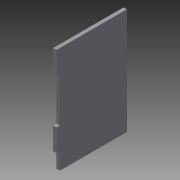
# Autodesk Inventor part: Motor support
Saved by Autodesk Inventor 2015 (Build 190159000, 159)
## iProperties
Created: 2014-11-11
Part Number: Motor support
Material: Generic
Document SubType Name: Modeling
Designer: karl
Density: 1 g/cm^3
Appearance: Default
Author: karl
Autodesk Inventor part; units mm, degrees
ref_plane "YZ Plane" through (0, 0, 0) normal (1, 0, 0) x (0, 1, 0)
ref_plane "XZ Plane" through (0, 0, 0) normal (0, 1, 0) x (-1, 0, 0)
ref_plane "XY Plane" through (0, 0, 0) normal (0, 0, 1) x (1, 0, 0)
sketch "Sketch1" plane through (0, 0, 0) normal (1, 0, 0) x (0, 1, 0)
  line L0 (-35, -47.5) -> (35, -47.5)
  line L1 (35, -47.5) -> (35, 47.5)
  line L2 (35, 47.5) -> (-35, 47.5)
  line L3 (-35, 47.5) -> (-35, -47.5)
  line L4 (-35, -47.5) -> (35, 47.5) construction
  line L5 (35, -47.5) -> (-35, 47.5) construction
  point P0 (0, 0)
  dimension "d0" = 70
  dimension "d1" = 95
  constraints: 12 end point, 2 midpoint, 2 parallel, 1 horizontal, 1 perpendicular
  measures "d0" distance of L2.end L1.end
  measures "d1" distance of L1.end L0.end
extrude "Extrusion1" add sketch "Sketch1" along normal blind 3
sketch "Sketch2" plane through (3, 0, 0) normal (1, 0, 0) x (0, 0, -1)
  line L0 (-47.5, -35) -> (47.5, -35) projected
  line L1 (32.5, -35) -> (12.5, -35)
  line L2 (12.5, -35) -> (12.5, -38)
  line L3 (12.5, -38) -> (32.5, -38)
  line L4 (32.5, -38) -> (32.5, -35)
  line L5 (-27.5, -35) -> (-47.5, -35)
  line L6 (-47.5, -35) -> (-47.5, -38)
  line L7 (-47.5, -38) -> (-27.5, -38)
  line L8 (-27.5, -38) -> (-27.5, -35)
  line L9 (47.5, -35) -> (47.5, 35) projected
  point P0 (0, 0)
  dimension "d4" = 20
  dimension "d5" = 3
  dimension "d6" = 20
  dimension "d7" = 3
  dimension "d8" = 40
  dimension "d9" = 15
  constraints: 16 end point, 4 parallel, 2 horizontal, 2 perpendicular, 2 point on line
  measures "d4" distance of L3.end L2.end
  measures "d5" distance of L2.end L1.end
  measures "d6" distance of L7.end L6.end
  measures "d7" distance of L6.end L5.end
  measures "d8" distance between parallel lines of L2 L8
  measures "d9" distance between parallel lines of L9 L4
extrude "Extrusion2" add sketch "Sketch2" against normal blind 3
sketch "Sketch3" plane through (3, 0, 0) normal (1, 0, 0) x (0, 0, -1)
  line L0 (47.5, -35) -> (47.5, 35) projected
  line L1 (47.5, 25) -> (50.5, 25)
  line L2 (50.5, 25) -> (50.5, 5)
  line L3 (50.5, 5) -> (47.5, 5)
  line L4 (47.5, 5) -> (47.5, 25)
  line L5 (47.5, 35) -> (-47.5, 35) projected
  line L6 (47.5, -15) -> (50.5, -15)
  line L7 (50.5, -15) -> (50.5, -25)
  line L8 (50.5, -25) -> (47.5, -25)
  line L9 (47.5, -25) -> (47.5, -15)
  line L10 (32.5, -35) -> (47.5, -35) projected
  point P0 (0, 0)
  dimension "d12" = 3
  dimension "d13" = 20
  dimension "d14" = 10
  dimension "d15" = 3
  dimension "d16" = 10
  dimension "d17" = 10
  dimension "d18" = 20
  constraints: 16 end point, 4 parallel, 2 horizontal, 2 perpendicular, 2 point on line
  measures "d12" distance of L2.end L3.end
  measures "d13" distance of L1.end L2.end
  measures "d14" distance between parallel lines of L5 L1
  measures "d15" distance of L7.end L8.end
  measures "d16" distance of L6.end L7.end
  measures "d17" distance between parallel lines of L10 L8
  measures "d18" distance between parallel lines of L3 L6
extrude "Extrusion3" add sketch "Sketch3" against normal blind 3
sketch "Sketch4" plane through (3, 0, 0) normal (1, 0, 0) x (0, 0, -1)
  line L0 (32.5, -35) -> (32.5, -38) projected
  line L1 (40.5, -38) -> (32.5, -38) projected
  line L2 (40.5, -35) -> (40.5, -38) projected
  line L3 (32.5, -35) -> (40.5, -35) projected
  line L4 (12.5, -38) -> (12.5, -35) projected
  line L5 (-19.5, -35) -> (12.5, -35) projected
  line L6 (-19.5, -35) -> (-19.5, -38) projected
  line L7 (12.5, -38) -> (-19.5, -38) projected
  circle A0 centre (10.5, -20) radius 30 construction
  circle A1 centre (10.5, -20) radius 2
  point P0 (0, 0)
  dimension "d21" = 60
  dimension "d22" = 30
  dimension "d23" = 15
  dimension "d24" = 4
  constraints: 2 centre point, 1 coincident
  measures "d21" diameter of A0
  measures "d22" distance from line of A0.centre L2
  measures "d23" distance from line of L5 A0.centre
  measures "d24" diameter of A1
extrude "Extrusion4" cut sketch "Sketch4" against normal blind 3 contours A1
sketch "Sketch5" plane through (3, 0, 0) normal (1, 0, 0) x (0, 0, -1)
  circle A0 centre (10.5, -15.5) radius 1
  circle A1 centre (10.5, -20) radius 2 projected
  circle A2 centre (6, -20) radius 1
  circle A3 centre (10.5, -24.5) radius 1
  circle A4 centre (15, -20) radius 1
  point P0 (0, 0)
  dimension "d27" = 2
  dimension "d28" = 4.5
  dimension "d31" = 360
  constraints: 4 centre point, 1 vertical alignment, 9 other
  measures "d27" diameter of A0
  measures "d28" distance of A1.centre A0.centre
extrude "Extrusion5" cut sketch "Sketch5" against normal blind 3 contours A0 | A2 | A3 | A4
body "Solid1"
